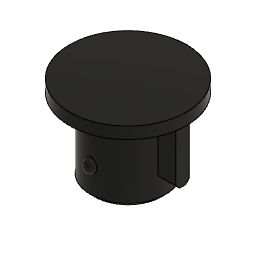
Pairing_Button_M3 (Autodesk Fusion 360 design; units mm, degrees)
Autodesk Fusion 360 part; units mm, degrees
note: some values were not read from the file. Chosen so that the rebuilt part matches the saved one: which sketch regions a step uses; where a step ends.
sketch "Skizze3" plane through (0, 0, 0) normal (1, 0, 0) x (0, 1, 0)
  line L0 (0, 0) -> (7.5, 0)
  line L1 (7.5, 0) -> (7.5, -1.5)
  line L2 (7.5, -1.5) -> (4.8, -3)
  line L3 (4.8, -3) -> (4.8, -11)
  line L4 (4.8, -11) -> (0, -11)
  line L5 (0, -11) -> (0, 0)
  dimension "d540" = 11
  dimension "d541" = 8
  dimension "d543" = 9.6
  dimension "d545" = 15
  dimension "d546" = 1.5
  constraint coincident L0.start L5.end
  constraint horizontal L0
  constraint perpendicular L0 L1
  constraint parallel L1 L3
  constraint perpendicular L3 L4
  constraint perpendicular L0 L5
  measures "d540" distance of L0 L4
  measures "d541" distance of L2.end L3.end
  measures "d546" distance of L0.end L1.end
revolve "Drehen1" add sketch "Skizze3" angle 360 about axis through (0, 0, -11) along (0, 0, 1) makes body 1
sketch "Skizze5" plane through (0, 0, -11) normal (0, 0, -1) x (1, 0, 0)
  circle A0 centre (0, 0) radius 4.8
  line L0 (-7, 0.875) -> (7, 0.875)
  line L1 (7, 0.875) -> (7, -0.875)
  line L2 (7, -0.875) -> (-7, -0.875)
  line L3 (-7, -0.875) -> (-7, 0.875)
  line L4 (-7, 0.875) -> (7, -0.875) construction
  line L5 (7, 0.875) -> (-7, -0.875) construction
  dimension "d565" = 1.75
  dimension "d566" = 14
  constraint horizontal L0
  constraint perpendicular L0 L1
  constraint parallel L0 L2
  constraint parallel L1 L3
  constraint coincident L4 A0.centre
  constraint coincident L5 A0.centre
  constraint coincident A0.centre origin
  measures "d565" distance of L0.start L2.end
  measures "d566" distance of L0.start L0.end
extrude "Extrusion3" add sketch "Skizze5" along normal up to near side of body 1 from surface at -2.5 contours A0 L0 L1 L2 | A0 L0 L2 L3 bodies 1
chamfer "Fase1" distance 0.5 angle 45 5 edges at (-4.4752, 1.7358, -11) (5.8598, -0.875, -8.5) (5.8598, 0.875, -8.5) (-5.8598, -0.875, -8.5) (-5.8598, 0.875, -8.5) on bodies 1
sketch "Skizze4" plane through (0, 0, -11) normal (0, 0, -1) x (1, 0, 0)
  circle A0 centre (0, 0) radius 4.3
  line L0 (2.5285, 0.3266) -> (1.3982, -0.8033)
  spline S0 degree 3 poles (1.3982, -0.8033) (0.7743, -1.4275) (-0.2377, -1.4275) (-0.8616, -0.8033) knots 0 0 0 0 1 1 1 1
  spline S1 degree 3 poles (-0.8616, -0.8033) (-0.9599, -0.7053) (-1.0368, -0.5949) (-1.1043, -0.481) knots 0 0 0 0 1 1 1 1
  line L1 (-1.1043, -0.481) -> (-0.5791, 0.0442)
  spline S2 degree 3 poles (-0.5791, 0.0442) (-0.5542, 0.0693) (-0.5233, 0.0838) (-0.4939, 0.1007) knots 0 0 0 0 1 1 1 1
  spline S3 degree 3 poles (-0.4939, 0.1007) (-0.4576, -0.0233) (-0.3942, -0.1408) (-0.2967, -0.2383) knots 0 0 0 0 1 1 1 1
  spline S4 degree 3 poles (-0.2967, -0.2383) (0.0149, -0.55) (0.5219, -0.5497) (0.8332, -0.2383) knots 0 0 0 0 1 1 1 1
  line L2 (0.8332, -0.2383) -> (1.9632, 0.8916)
  spline S5 degree 3 poles (1.9632, 0.8916) (2.2749, 1.2033) (2.2749, 1.7102) (1.9632, 2.0217) knots 0 0 0 0 1 1 1 1
  spline S6 degree 3 poles (1.9632, 2.0217) (1.6518, 2.3333) (1.145, 2.3333) (0.8332, 2.0217) knots 0 0 0 0 1 1 1 1
  line L3 (0.8332, 2.0217) -> (0.4314, 1.6195)
  spline S7 degree 3 poles (0.4314, 1.6195) (0.1054, 1.7464) (-0.2459, 1.7806) (-0.5879, 1.7305) knots 0 0 0 0 1 1 1 1
  line L4 (-0.5879, 1.7305) -> (0.2683, 2.5867)
  spline S8 degree 3 poles (0.2683, 2.5867) (0.8925, 3.2107) (1.9042, 3.2107) (2.5285, 2.5867) knots 0 0 0 0 1 1 1 1
  spline S9 degree 3 poles (2.5285, 2.5867) (3.1524, 1.9626) (3.1524, 0.9507) (2.5285, 0.3266) knots 0 0 0 0 1 1 1 1
  line L5 (-0.4596, -1.5313) -> (-0.8616, -1.9336)
  spline S10 degree 3 poles (-0.8616, -1.9336) (-1.1732, -2.2449) (-1.6802, -2.2449) (-1.9917, -1.9336) knots 0 0 0 0 1 1 1 1
  spline S11 degree 3 poles (-1.9917, -1.9336) (-2.3033, -1.6218) (-2.3033, -1.115) (-1.9917, -0.8033) knots 0 0 0 0 1 1 1 1
  line L6 (-1.9917, -0.8033) -> (-0.8616, 0.3266)
  spline S12 degree 3 poles (-0.8616, 0.3266) (-0.5499, 0.6384) (-0.0433, 0.6384) (0.2683, 0.3266) knots 0 0 0 0 1 1 1 1
  spline S13 degree 3 poles (0.2683, 0.3266) (0.3656, 0.2293) (0.429, 0.1118) (0.4657, -0.012) knots 0 0 0 0 1 1 1 1
  spline S14 degree 3 poles (0.4657, -0.012) (0.4954, 0.0051) (0.5258, 0.0192) (0.5508, 0.0441) knots 0 0 0 0 1 1 1 1
  line L7 (0.5508, 0.0441) -> (1.0759, 0.5691)
  spline S15 degree 3 poles (1.0759, 0.5691) (1.0088, 0.6834) (0.9316, 0.7935) (0.8333, 0.8916) knots 0 0 0 0 1 1 1 1
  spline S16 degree 3 poles (0.8333, 0.8916) (0.2094, 1.5156) (-0.8027, 1.5156) (-1.4268, 0.8916) knots 0 0 0 0 1 1 1 1
  line L8 (-1.4268, 0.8916) -> (-2.5567, -0.2383)
  spline S17 degree 3 poles (-2.5567, -0.2383) (-3.1807, -0.8626) (-3.1807, -1.8743) (-2.5567, -2.4985) knots 0 0 0 0 1 1 1 1
  spline S18 degree 3 poles (-2.5567, -2.4985) (-1.9326, -3.1224) (-0.9207, -3.1224) (-0.2967, -2.4985) knots 0 0 0 0 1 1 1 1
  line L9 (-0.2967, -2.4985) -> (0.5598, -1.6421)
  spline S19 degree 3 poles (0.5598, -1.6421) (0.2176, -1.6925) (-0.1338, -1.6581) (-0.4596, -1.5313) knots 0 0 0 0 1 1 1 1
extrude "Extrusion2" cut sketch "Skizze4" against normal blind 0.5 contours L0 S0 S1 L1 S2 S3 S4 L2 S5 S6 L3 S7 L4 S8 S9 | L5 S10 S11 L6 S12 S13 S14 L7 S15 S16 L8 S17 S18 L9 S19 bodies 1
extrude "Extrusion1" add 2 faces at (-1.4267, -0.1383, -10.5) (1.9633, -0.1383, -10.5) along direction (0, 0, -1) blind 0.5 separate body on bodies 1 makes body 2 at (-1.4267, -0.1383, -10.5) makes body 3 at (1.9633, -0.1383, -10.5) in component "Pairing_Button_Text"
sketch "Skizze6" plane through (0, 0, 0) normal (1, 0, 0) x (0, 1, 0)
  line L0 (0.875, -8) -> (0.875, -3)
  line L1 (0.875, -3) -> (4.8, -3)
  line L2 (0.875, -3) -> (0.875, -8)
  line L3 (0.875, -8) -> (0.375, -8.5)
  line L4 (-0.375, -8.5) -> (0.375, -8.5)
  line L5 (-0.375, -8.5) -> (-0.875, -8)
  line L6 (-0.875, -8) -> (-0.875, -3)
  line L7 (-4.8, -3) -> (-0.875, -3)
  line L8 (-0.875, -3) -> (-0.875, -8)
  line L9 (-0.375, -8.5) -> (-0.875, -8)
  line L10 (-0.375, -8.5) -> (0.375, -8.5)
  line L11 (0.875, -8) -> (0.375, -8.5)
  line L12 (-4.8, -10.5) -> (4.8, -10.5)
  line L13 (-4.8, -3.5) -> (-4.8, -11)
  circle A0 centre (-4.55, -7.25) radius 1
  point P0 (-4.8, -7.25)
  dimension "d581" = 2
  dimension "d582" = 0.25
  constraint midpoint L13 P0
  constraint horizontal A0.centre P0
  measures "d581" diameter of A0
  measures "d582" distance of L13 A0.centre
revolve "Drehen2" add sketch "Skizze6" angle 360 about axis through (0, -4.8, -3.5) along (0, 0, -1) contours L13 A0 picked at (-5.0464, -7.2986) bodies 1
component "Pairing_Button_Text" placed x (1, 0, 0) y (0, 1, 0) z (0, 0, 1) at (0, 0, 0)
equation "d543 = 10 mm - ( 2 * 0.2 ) * 1 mm"
equation "d565 = 2 mm - 0.25 mm"
equation "d566 = 10 mm + ( 2 * 2 ) * 1 mm"
equation "d582 = ( d581 / 2 ) - 0.75 mm"
named bodies: "Pairing_Button", "Pairing_Button_Text_1", "Pairing_Button_Text_2"
